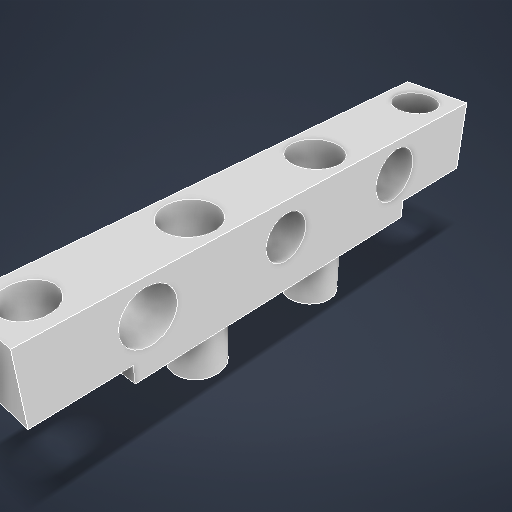
# Autodesk Inventor part: diff_gear_holder_4
Saved by Autodesk Inventor 2025 (Build 290162000, 162)
## iProperties
Created: 2024-07-25
Part Number: diff_gear_holder_4
Material: Generic
Document SubType Name: Modeling
Designer: Garfieldcmix
Density: 1 g/cm^3
Appearance: Default
Author: Garfieldcmix
Autodesk Inventor part; units mm, degrees
ref_plane "YZ Plane" through (0, 0, 0) normal (1, 0, 0) x (0, 1, 0)
ref_plane "XZ Plane" through (0, 0, 0) normal (0, 1, 0) x (-1, 0, 0)
ref_plane "XY Plane" through (0, 0, 0) normal (0, 0, 1) x (1, 0, 0)
sketch "Sketch1" plane through (0, 0, 0) normal (0, 1, 0) x (-1, 0, 0)
  line L0 (0, 0) -> (7.8, 0)
  line L1 (7.8, 0) -> (7.8, -55.8)
  line L2 (7.8, -55.8) -> (0, -55.8)
  line L3 (0, -55.8) -> (0, 0)
  line L4 (3.9, 0) -> (3.9, -55.8) construction
  line L5 (7.8, -27.9) -> (0, -27.9) construction
  circle A0 centre (3.9, -19.9) radius 3
  circle A1 centre (3.9, -19.9) radius 1.5
  circle A2 centre (3.9, -35.9) radius 3
  circle A3 centre (3.9, -35.9) radius 1.5
  circle A4 centre (3.9, -3.9) radius 2.4
  circle A5 centre (3.9, -51.9) radius 2.4
  line L6 (0, -9.9) -> (7.8, -9.9)
  line L7 (0, -45.9) -> (7.8, -45.9)
  dimension "d0" = 7.8
  dimension "d1" = 55.8
  dimension "d3" = 6
  dimension "d4" = 3
  dimension "d25" = 8
  dimension "d26" = 4.8
  dimension "d27" = 16
  dimension "d28" = 18
  constraints: 16 end point, 6 centre point, 5 symmetric about line, 4 coincident, 4 midpoint, 4 point on line, 2 parallel, 2 perpendicular, 1 horizontal, 3 other
  measures "d0" distance of L1.end L2.end
  measures "d1" distance of L0.end L1.end
  measures "d3" diameter of A0
  measures "d4" diameter of A1
  measures "d25" distance from line of L5 point (3.9, -19.9)
  measures "d26" diameter of A4
  measures "d27" distance of point (3.9, -19.9) point (3.9, -3.9)
  measures "d28" distance between parallel lines of L5 L6
extrude "Extrusion1" add sketch "Sketch1" along normal blind 8 contours L0 L1 L6 L3 | L6 L1 L7 L3 | L7 L1 L2 L3
extrude "Extrusion2" add sketch "Sketch1" against normal blind 2 contours L6 L1 L7 L3 | A0 | A2
extrude "Extrusion3" add sketch "Sketch1" against normal blind 6 from surface at -2 contours A0 | A2
sketch "Sketch2" plane through (0, 8, 0) normal (1, 0, 0) x (0, 0, -1)
  line L0 (0, 0) -> (55.8, 0) construction
  line L1 (0, -8) -> (0, 0) construction
  line L2 (45.9, -10) -> (9.9, -10) construction
  line L3 (55.8, 0) -> (55.8, -10) construction
  line L4 (27.9, 0) -> (27.9, -10) construction
  line L5 (9.9, -10) -> (45.9, -10) construction
  circle A0 centre (27.9, -4) radius 2.4
  line L6 (55.8, 0) -> (0, 0) projected
  line L7 (11.9, 0) -> (11.9, -10) construction
  circle A1 centre (11.9, -4) radius 1.5
  circle A2 centre (11.9, -4) radius 3
  circle A3 centre (43.9, -4) radius 1.5
  circle A4 centre (43.9, -4) radius 3
  point P0 (0, -10)
  dimension "d11" = 4
  dimension "d12" = 4.8
  dimension "d17" = 4
  dimension "d18" = 3
  dimension "d19" = 6
  dimension "d22" = 16
  constraints: 5 centre point, 4 coincident, 4 end point, 4 point on line, 2 midpoint, 2 symmetric about line, 1 perpendicular, 2 other
  measures "d11" distance from line of L0 point (27.9, -4)
  measures "d12" diameter of A0
  measures "d17" distance from line of point (11.9, -4) L0
  measures "d18" diameter of A1
  measures "d19" diameter of A2
  measures "d22" distance between parallel lines of L7 L4
extrude "Extrusion4" cut sketch "Sketch2" against normal through all contours A0
extrude "Extrusion5" cut sketch "Sketch2" against normal blind 6 contours A1 | A2 | A3 | A4
extrude "Extrusion6" cut sketch "Sketch2" against normal through all contours A1 | A3
offset faces "Size1" outward -0.21 faces at (-2.6, 3.615, -30.2689)
offset faces "Size2" outward -0.06 faces at (-3.9964, 0, -47.1058) (-3.9964, 0, -8.6942)
offset faces "Size3" outward -0.16 faces at (-6.2922, 2.7067, -51.7069) (-6.2922, 2.7067, -3.7069)
body "Solid1"
